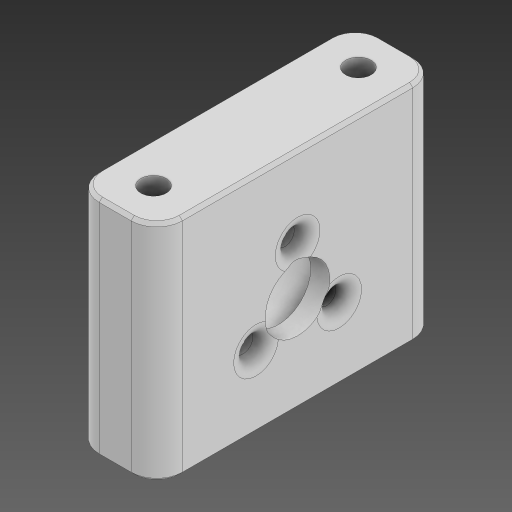
# Autodesk Inventor part: fastenin_motor
Saved by Autodesk Inventor 2023 (Build 270158000, 158)
## iProperties
Created: 2025-06-22
Part Number: fastenin_motor
Material: Типовые
Document SubType Name: Modeling
Designer: daa
Density: 1 g/cm^3
Appearance: По умолчанию
Author: daa
Autodesk Inventor part; units mm, degrees
ref_plane "YZ Plane" through (0, 0, 0) normal (1, 0, 0) x (0, 1, 0)
ref_plane "XZ Plane" through (0, 0, 0) normal (0, 1, 0) x (-1, 0, 0)
ref_plane "XY Plane" through (0, 0, 0) normal (0, 0, 1) x (1, 0, 0)
sketch "Эскиз1" plane through (0, 0, 0) normal (0, 1, 0) x (-1, 0, 0)
  line L0 (4, 13) -> (-1, 13)
  line L1 (-5, 9) -> (-5, -27)
  line L2 (-1, -31) -> (4, -31)
  line L3 (8, -27) -> (8, 9)
  circle A0 centre (1.5, 7) radius 2
  circle A1 centre (1.5, -25) radius 2
  arc A2 (8, 9) -> (4, 13) centre (4, 9) ccw
  arc A3 (-1, 13) -> (-5, 9) centre (-1, 9) ccw
  arc A4 (-5, -27) -> (-1, -31) centre (-1, -27) ccw
  arc A5 (4, -31) -> (8, -27) centre (4, -27) ccw
  point P0 (0, 0)
  point P1 (-5, -31)
  point P2 (-5, 13)
  point P3 (8, -31)
  dimension "d0" = 13
  dimension "d1" = 44
  dimension "d2" = 4
  dimension "d3" = 4
  dimension "d4" = 32
  dimension "d5" = 6.5
  dimension "d6" = 6
  dimension "d7" = 4
  constraints: 8 end point, 8 point on circle, 8 tangent, 6 centre point, 6 point on line, 3 equal radius, 2 parallel, 1 horizontal, 1 perpendicular
  measures "d0" distance of point (8, -31) point (-5, -31)
  measures "d1" distance of point (-5, -31) point (-5, 13)
  measures "d2" diameter of A0
  measures "d3" diameter of A1
  measures "d4" distance of A1.centre A0.centre
  measures "d5" distance from line of L1 A0.centre
  measures "d6" distance from line of A0.centre L0
  measures "d7" radius of A2
extrude "Выдавливание1" add sketch "Эскиз1" along normal blind 35
sketch "Эскиз2" plane through (-8, 0, -27) normal (-1, 0, 0) x (0, 0, 1)
  circle A0 centre (18, 15) radius 10.1
  circle A1 centre (18, 15) radius 5.05
  line L0 (0, 0) -> (36, 0) projected
  line L1 (36, 0) -> (36, 35) projected
  circle A2 centre (18, 15) radius 7.5 construction
  circle A3 centre (18, 22.5) radius 1.5
  line L2 (18, 15) -> (25.5, 15)
  line L3 (18, 15) -> (24.4952, 11.25)
  line L4 (18, 15) -> (25.5, 15) construction
  circle A4 centre (24.4952, 11.25) radius 1.5
  line L5 (18, 15) -> (10.5, 15)
  line L6 (18, 15) -> (24.4952, 11.25)
  line L7 (18, 15) -> (25.5, 15) construction
  line L8 (18, 15) -> (11.5048, 11.25)
  line L9 (18, 15) -> (25.5, 15) construction
  circle A5 centre (11.5048, 11.25) radius 1.5
  point P0 (27, 0)
  dimension "d10" = 20.2
  dimension "d11" = 10.1
  dimension "d12" = 15
  dimension "d13" = 18
  dimension "d14" = 15
  dimension "d15" = 3
  dimension "d16" = 30
  dimension "d17" = 3
  dimension "d18" = 30
  dimension "d19" = 150
  dimension "d20" = 3
  constraints: 16 end point, 6 centre point, 5 horizontal, 5 point on circle, 4 coincident, 3 equal length
  measures "d10" diameter of A0
  measures "d11" diameter of A1
  measures "d12" distance from line of L0 A0.centre
  measures "d13" distance from line of L1 A0.centre
  measures "d14" diameter of A2
  measures "d15" diameter of A3
  measures "d16" angle of L3 L4
  measures "d17" diameter of A4
  measures "d18" angle of L6 L7
  measures "d19" angle of L8 L9
  measures "d20" diameter of A5
extrude "Выдавливание2" cut sketch "Эскиз2" against normal blind 40 contours L2 L5 A1 | A1 L3 L2 | L5 L8 A1 | A1 L8 L3 | A3 | A4 | A5
sketch "Эскиз3" plane through (-8, 0, -27) normal (-1, 0, 0) x (0, 0, 1)
  circle A0 centre (18, 15) radius 5
  circle A1 centre (18, 15) radius 10.1
  line L0 (0, 0) -> (36, 0) projected
  point P0 (27, 0)
  dimension "d23" = 20.2
  dimension "d29" = 15
  constraints: 2 centre point, 1 coincident
  measures "d23" diameter of A1
  measures "d29" distance from line of L0 A0.centre
extrude "Выдавливание3" cut sketch "Эскиз3" against normal blind 10
chamfer "Фаска1" distance 0.5 angle 45 16 edges at (-8, 35, -9) (-6.8284, 35, 11.8284) (-1.5, 35, 13) (3.8284, 35, 11.8284) (5, 35, -9) (3.8284, 35, -29.8284) (-1.5, 35, -31) (-6.8284, 35, -29.8284) (-8, 0, -9) (-6.8284, 0, 11.8284) (-1.5, 0, 13) (3.8284, 0, 11.8284) (5, 0, -9) (3.8284, 0, -29.8284) (-1.5, 0, -31) (-6.8284, 0, -29.8284)
fillet "Сопряжение1" radius 2 3 edges at (5, 22.5, -10.5) (5, 11.25, -4.0048) (5, 11.25, -16.9952)
